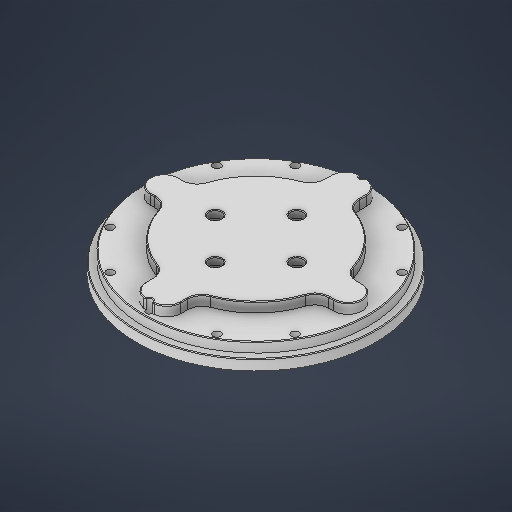
# Autodesk Inventor part: Build Plateform
Saved by Autodesk Inventor 2025 (Build 290162000, 162)
## iProperties
Created: 2024-08-23
Part Number: Build Plateform
Material: Generic
Document SubType Name: Modeling
Designer: mayhe
Density: 1 g/cm^3
Appearance: Default
Author: mayhe
Autodesk Inventor part; units mm, degrees
ref_plane "YZ Plane" through (0, 0, 0) normal (1, 0, 0) x (0, 1, 0)
ref_plane "XZ Plane" through (0, 0, 0) normal (0, 1, 0) x (-1, 0, 0)
ref_plane "XY Plane" through (0, 0, 0) normal (0, 0, 1) x (1, 0, 0)
sketch "Sketch1" plane through (0, 0, 0) normal (0, 1, 0) x (-1, 0, 0)
  circle A0 centre (0, 0) radius 85
  circle A1 centre (0, 0) radius 80
  circle A2 centre (0, 0) radius 76
  line L0 (65, 0) -> (65, 0)
  line L1 (-2.5, -76) -> (2.5, -76)
  line L2 (2.5, 76) -> (-2.5, 76)
  line L3 (-12.5, -76) -> (12.5, 76) construction
  line L4 (12.5, -76) -> (-12.5, 76) construction
  line L5 (-75.339233, 0) -> (-75.339233, 0)
  line L6 (75.339233, 0) -> (75.339233, 0)
  line L7 (75.339233, 10) -> (-75.339233, -10) construction
  line L8 (-75.339233, 10) -> (75.339233, -10) construction
  arc A3 (65.339233, -10) -> (75.339233, 0) centre (65.339233, 0) ccw
  arc A4 (75.339233, 0) -> (65.339233, 10) centre (65.339233, 0) ccw
  arc A5 (12.5, 66) -> (2.5, 76) centre (2.5, 66) ccw
  arc A6 (-2.5, 76) -> (-12.5, 66) centre (-2.5, 66) ccw
  arc A7 (2.5, -76) -> (12.5, -66) centre (2.5, -66) ccw
  arc A8 (-12.5, -66) -> (-2.5, -76) centre (-2.5, -66) ccw
  arc A9 (-75.339233, 0) -> (-65.339233, -10) centre (-65.339233, 0) ccw
  arc A10 (-65.339233, 10) -> (-75.339233, 0) centre (-65.339233, 0) ccw
  arc A11 (-52.331725, -16.923077) -> (-19.038462, -51.599777) centre (0, 0) ccw
  arc A12 (19.038462, -51.599777) -> (52.331725, -16.923077) centre (0, 0) ccw
  arc A13 (52.331725, 16.923077) -> (19.038462, 51.599777) centre (0, 0) ccw
  arc A14 (-19.038462, 51.599777) -> (-52.331725, 16.923077) centre (0, 0) ccw
  line L9 (12.5, -66) -> (12.5, -60.981555)
  line L10 (12.5, -1.659162) -> (12.5, 1.659162)
  line L11 (12.5, 60.981555) -> (12.5, 66)
  line L12 (-12.5, 66) -> (-12.5, 60.981555)
  line L13 (-12.5, -60.981555) -> (-12.5, -66)
  line L14 (-65.339233, -10) -> (-61.846584, -10)
  line L15 (61.846584, -10) -> (65.339233, -10)
  line L16 (65.339233, 10) -> (61.846584, 10)
  line L17 (-61.846584, 10) -> (-65.339233, 10)
  arc A15 (-12.5, -60.981555) -> (-19.038462, -51.599777) centre (-22.5, -60.981555) ccw
  arc A16 (-52.331725, -16.923077) -> (-61.846584, -10) centre (-61.846584, -20) ccw
  arc A17 (-61.846584, 10) -> (-52.331725, 16.923077) centre (-61.846584, 20) ccw
  arc A18 (-19.038462, 51.599777) -> (-12.5, 60.981555) centre (-22.5, 60.981555) ccw
  arc A19 (12.5, 60.981555) -> (19.038462, 51.599777) centre (22.5, 60.981555) ccw
  arc A20 (52.331725, 16.923077) -> (61.846584, 10) centre (61.846584, 20) ccw
  arc A21 (61.846584, -10) -> (52.331725, -16.923077) centre (61.846584, -20) ccw
  arc A22 (19.038462, -51.599777) -> (12.5, -60.981555) centre (22.5, -60.981555) ccw
  point P0 (-54.083269, 10)
  point P1 (-54.083269, -10)
  point P2 (-12.5, -53.560713)
  point P3 (12.5, -53.560713)
  point P4 (54.083269, -10)
  point P5 (54.083269, 10)
  point P6 (12.5, 53.560713)
  point P7 (-12.5, 53.560713)
  point P8 (3.918132, 75.898934)
  point P9 (-3.918132, 75.898934)
  point P10 (-3.918132, -75.898934)
  point P11 (3.918132, -75.898934)
  point P12 (75.339233, 0)
  point P13 (0, -76)
  point P14 (0, 76)
  dimension "d26" = 152
  dimension "d24" = 170
  dimension "d25" = 160
  dimension "d27" = 25
  dimension "d29" = 20
  dimension "d30" = 10
  dimension "d31" = 10
  dimension "d32" = 10
  constraints: 48 point on circle, 42 tangent, 36 end point, 22 centre point, 18 point on line, 13 equal radius, 12 parallel, 5 perpendicular, 4 midpoint, 3 coincident, 3 horizontal, 3 other
  measures "d24" diameter of A0
  measures "d25" diameter of A1
  measures "d27" distance of L4.end L3.end
  measures "d29" distance of L7.end L8.start
  measures "d30" radius of A3
  measures "d31" radius of A15
  measures "d32" radius of A18
extrude "Extrusion1" add sketch "Sketch1" along normal blind 21.5 contours A5 L11 A19 A13 A20 L16 A4 A3 L15 A21 A12 A22 L9 A7 A2 A8 L13 A15 A11 A16 L14 A9 A10 L17 A17 A14 A18 L12 A6
extrude "Extrusion2" add sketch "Sketch1" along normal blind 14.5 contours A1 | A2 A7 L9 A22 A12 A21 L15 A3 A4 L16 A20 A13 A19 L11 A5 | A2 L2 A5 | A7 L1 A2 | A2 A6 L2 | L1 A8 A2 | A6 L12 A18 A14 A17 L17 A10 A9 L14 A16 A11 A15 L13 A8 A2
extrude "Extrusion3" add sketch "Sketch1" along normal blind 7.5 contours A0
sketch "Sketch2" plane through (0, 21.5, 0) normal (0, 1, 0) x (1, 0, 0)
  circle A0 centre (0, 0) radius 29
  circle A1 centre (0, 29) radius 4.5
  circle A2 centre (0, 29) radius 2.5
  circle A3 centre (-29, 0) radius 4.5
  circle A4 centre (-29, 0) radius 2.5
  circle A5 centre (0, -29) radius 4.5
  circle A6 centre (0, -29) radius 2.5
  circle A7 centre (29, 0) radius 4.5
  circle A8 centre (29, 0) radius 2.5
  dimension "d40" = 58
  dimension "d41" = 9
  dimension "d42" = 5
  dimension "d45" = 360
  constraints: 8 centre point, 5 coincident, 1 vertical alignment, 19 other
  measures "d41" diameter of A1
  measures "d42" diameter of A2
extrude "Extrusion4" cut sketch "Sketch2" against normal blind 5 contours A0 A8 | A0 A8 | A8 A0 A7 | A0 A7 A8 | A1 A0 A2 | A0 A2 A1 | A5 A0 A6 | A0 A6 A5 | A2 A0 | A0 A2 | A6 A0 | A0 A6 | A3 A0 A4 | A0 A4 A3 | A4 A0 | A0 A4
hole "Hole1" at (29, 21.5, 0) at (0, 21.5, 29) at (-29, 21.5, 0) at (0, 21.5, -29) direction (0, -1, 0) diameter 5.5 end through all
sketch "Sketch3" plane through (0, 21.5, 0) normal (0, 1, 0) x (1, 0, 0)
  circle A0 centre (0, 0) radius 76
  circle A1 centre (0, 76) radius 1.75
  circle A2 centre (0, -76) radius 1.75
  dimension "d56" = 152
  dimension "d57" = 3.5
  dimension "d60" = 360
  constraints: 2 centre point, 1 coincident, 1 vertical alignment, 7 other
  measures "d57" diameter of A1
hole "Hole2" at (0, 21.5, -76) at (0, 21.5, 76) direction (0, -1, 0) diameter 4.5 end through all
sketch "Sketch4" plane through (0, 0, 0) normal (0, -1, 0) x (1, 0, 0)
  arc A0 (-19.364917, 35) -> (19.364917, 35) centre (0, 0) ccw
  line L0 (19.364917, 35) -> (-19.364917, 35)
  circle A1 centre (0, 0) radius 10
  dimension "d69" = 80
  dimension "d70" = 5
  dimension "d71" = 20
  constraints: 2 centre point, 2 coincident, 2 end point, 2 point on circle, 1 horizontal
  measures "d69" diameter of A0
  measures "d70" distance edge to line of A0 L0
  measures "d71" diameter of A1
extrude "Extrusion5" cut sketch "Sketch4" against normal blind 1.5
extrude "Extrusion6" cut sketch "Sketch4" against normal blind 12 contours A1
sketch "Sketch5" plane through (0, 14.5, 0) normal (0, 1, 0) x (1, 0, 0)
  circle A0 centre (0, 0) radius 10
  arc A1 (-2.249753, 75.966694) -> (2.249753, 75.966694) centre (0, 76) ccw
  circle A2 centre (0, 0) radius 76
  arc A3 (2.249753, -75.966694) -> (-2.249753, -75.966694) centre (0, -76) ccw
  circle A4 centre (0, -76) radius 2.5
  circle A5 centre (38, -65.817931) radius 2.5
  circle A6 centre (65.817931, -38) radius 2.5
  circle A7 centre (76, 0) radius 2.5
  circle A8 centre (65.817931, 38) radius 2.5
  circle A9 centre (38, 65.817931) radius 2.5
  circle A10 centre (0, 76) radius 2.5
  circle A11 centre (-38, 65.817931) radius 2.5
  circle A12 centre (-65.817931, 38) radius 2.5
  circle A13 centre (-76, 0) radius 2.5
  circle A14 centre (-65.817931, -38) radius 2.5
  circle A15 centre (-38, -65.817931) radius 2.5
  dimension "d76" = 5
  dimension "d79" = 360
  constraints: 13 centre point, 2 coincident, 1 point on circle, 25 other
  measures "d76" diameter of A4
hole "Hole3" at (-38, 14.5, 65.817931) at (-65.817931, 14.5, 38) at (-65.817931, 14.5, -38) at (-38, 14.5, -65.817931) at (38, 14.5, -65.817931) at (65.817931, 14.5, -38) at (65.817931, 14.5, 38) at (38, 14.5, 65.817931) direction (0, -1, 0) diameter 5.5 end through all
chamfer "Chamfer1" distance 0.5 angle 45 33 edges at (39.6742, 21.5, 38.0914) (55.9631, 21.5, 11.9139) (63.5929, 21.5, 10) (75.3392, 21.5, 0) (63.5929, 21.5, -10) (55.9631, 21.5, -11.9139) (39.6742, 21.5, -38.0914) (14.2959, 21.5, -55.2638) (12.5, 21.5, -63.4908) (10.0558, 21.5, -72.5505) (14.2959, 21.5, 55.2638) (12.5, 21.5, 63.4908) (10.0558, 21.5, 72.5505) (-14.2959, 21.5, 55.2638) (-12.5, 21.5, 63.4908) (-10.0558, 21.5, 72.5505) (-39.6742, 21.5, 38.0914) (-55.9631, 21.5, 11.9139) (-63.5929, 21.5, 10) (-75.3392, 21.5, 0) (-63.5929, 21.5, -10) (-55.9631, 21.5, -11.9139) (-39.6742, 21.5, -38.0914) (-14.2959, 21.5, -55.2638) (-12.5, 21.5, -63.4908) (-10.0558, 21.5, -72.5505) (-4.5, 21.5, 29) (-33.5, 21.5, 0) (-4.5, 21.5, -29) (24.5, 21.5, 0) (1.5792, 21.5, -74.3973) (-1.5792, 21.5, -74.3973) (0, 21.5, 73.75)
chamfer "Chamfer2" distance 0.5 angle 45 2 edges at (80, 14.5, 0) (85, 7.5, 0)
sketch "Sketch7" plane through (0, 21.5, 0) normal (0, 1, 0) x (1, 0, 0)
  circle A0 centre (0, 0) radius 47.5
  circle A1 centre (47.5, 0) radius 2.5
  circle A2 centre (43.884278, 18.177463) radius 2.5
  circle A3 centre (33.587572, 33.587572) radius 2.5
  circle A4 centre (18.177463, 43.884278) radius 2.5
  circle A5 centre (0, 47.5) radius 2.5
  circle A6 centre (-18.177463, 43.884278) radius 2.5
  circle A7 centre (-33.587572, 33.587572) radius 2.5
  circle A8 centre (-43.884278, 18.177463) radius 2.5
  circle A9 centre (-47.5, 0) radius 2.5
  circle A10 centre (-43.884278, -18.177463) radius 2.5
  circle A11 centre (-33.587572, -33.587572) radius 2.5
  circle A12 centre (-18.177463, -43.884278) radius 2.5
  circle A13 centre (0, -47.5) radius 2.5
  circle A14 centre (18.177463, -43.884278) radius 2.5
  circle A15 centre (33.587572, -33.587572) radius 2.5
  circle A16 centre (43.884278, -18.177463) radius 2.5
  dimension "d107" = 95
  dimension "d108" = 5
  dimension "d111" = 360
  constraints: 16 centre point, 1 coincident, 1 horizontal alignment, 35 other
  measures "d108" diameter of A1
hole "Hole5" [suppressed]
sketch "Sketch8" plane through (0, 0, 0) normal (0, -1, 0) x (1, 0, 0)
  circle A0 centre (38, -65.817931) radius 2.75
  circle A1 centre (0, -29) radius 2.75
  circle A2 centre (38, 65.817931) radius 2.75
  circle A3 centre (38, 65.817931) radius 3.875
  circle A4 centre (65.817931, 38) radius 2.75
  circle A5 centre (65.817931, 38) radius 3.875
  circle A6 centre (65.817931, -38) radius 2.75
  circle A7 centre (65.817931, -38) radius 3.875
  circle A8 centre (38, -65.817931) radius 3.875
  circle A9 centre (0, -76) radius 2.25
  circle A10 centre (-38, -65.817931) radius 2.75
  circle A11 centre (-38, -65.817931) radius 3.875
  circle A12 centre (-65.817931, -38) radius 2.75
  circle A13 centre (-65.817931, -38) radius 3.875
  circle A14 centre (-65.817931, 38) radius 2.75
  circle A15 centre (-65.817931, 38) radius 3.875
  circle A16 centre (-38, 65.817931) radius 2.75
  circle A17 centre (-38, 65.817931) radius 3.875
  circle A18 centre (29, 0) radius 2.75
  circle A19 centre (29, 0) radius 3.875
  circle A20 centre (0, -29) radius 3.875
  circle A21 centre (-29, 0) radius 2.75
  circle A22 centre (-29, 0) radius 3.875
  circle A23 centre (0, 29) radius 2.75
  circle A24 centre (0, 29) radius 3.875
  circle A25 centre (0, 76) radius 2.25
  circle A26 centre (0, 76) radius 3.625
  circle A27 centre (0, -76) radius 3.625
  line L0 (69.705483, 35.784651) -> (65.843159, 33.525607)
  line L1 (65.843159, 33.525607) -> (61.955606, 35.740955)
  line L2 (61.955606, 35.740955) -> (61.930378, 40.215349)
  line L3 (61.930378, 40.215349) -> (65.792703, 42.474393)
  line L4 (65.792703, 42.474393) -> (69.680255, 40.259045)
  line L5 (69.680255, 40.259045) -> (69.705483, 35.784651)
  line L6 (61.943019, -35.762615) -> (65.818107, -33.525535)
  line L7 (65.818107, -33.525535) -> (69.693019, -35.76292)
  line L8 (69.693019, -35.76292) -> (69.692843, -40.237385)
  line L9 (69.692843, -40.237385) -> (65.817755, -42.474465)
  line L10 (65.817755, -42.474465) -> (61.942843, -40.23708)
  line L11 (61.942843, -40.23708) -> (61.943019, -35.762615)
  line L12 (34.125, -63.580698) -> (38, -61.343466)
  line L13 (38, -61.343466) -> (41.875, -63.580698)
  line L14 (41.875, -63.580698) -> (41.875, -68.055163)
  line L15 (41.875, -68.055163) -> (38, -70.292395)
  line L16 (38, -70.292395) -> (34.125, -68.055163)
  line L17 (34.125, -68.055163) -> (34.125, -63.580698)
  line L18 (-3.606269, -73.874992) -> (0.037176, -71.814376)
  line L19 (0.037176, -71.814376) -> (3.643445, -73.939384)
  line L20 (3.643445, -73.939384) -> (3.606269, -78.125008)
  line L21 (3.606269, -78.125008) -> (-0.037176, -80.185624)
  line L22 (-0.037176, -80.185624) -> (-3.643445, -78.060616)
  line L23 (-3.643445, -78.060616) -> (-3.606269, -73.874992)
  line L24 (-41.875, -63.580698) -> (-38, -61.343466)
  line L25 (-38, -61.343466) -> (-34.125, -63.580698)
  line L26 (-34.125, -63.580698) -> (-34.125, -68.055163)
  line L27 (-34.125, -68.055163) -> (-38, -70.292395)
  line L28 (-38, -70.292395) -> (-41.875, -68.055163)
  line L29 (-41.875, -68.055163) -> (-41.875, -63.580698)
  line L30 (-69.692845, -35.76262) -> (-65.81776, -33.525535)
  line L31 (-65.81776, -33.525535) -> (-61.942845, -35.762916)
  line L32 (-61.942845, -35.762916) -> (-61.943016, -40.23738)
  line L33 (-61.943016, -40.23738) -> (-65.818101, -42.474465)
  line L34 (-65.818101, -42.474465) -> (-69.693016, -40.237084)
  line L35 (-69.693016, -40.237084) -> (-69.692845, -35.76262)
  line L36 (-69.776476, 40.085846) -> (-65.990807, 42.471124)
  line L37 (-65.990807, 42.471124) -> (-62.032262, 40.385278)
  line L38 (-62.032262, 40.385278) -> (-61.859386, 35.914154)
  line L39 (-61.859386, 35.914154) -> (-65.645054, 33.528876)
  line L40 (-65.645054, 33.528876) -> (-69.603599, 35.614722)
  line L41 (-69.603599, 35.614722) -> (-69.776476, 40.085846)
  line L42 (-41.875, 68.055163) -> (-38, 70.292395)
  line L43 (-38, 70.292395) -> (-34.125, 68.055163)
  line L44 (-34.125, 68.055163) -> (-34.125, 63.580698)
  line L45 (-34.125, 63.580698) -> (-38, 61.343466)
  line L46 (-38, 61.343466) -> (-41.875, 63.580698)
  line L47 (-41.875, 63.580698) -> (-41.875, 68.055163)
  line L48 (-3.675534, 78.002819) -> (-0.103274, 80.184515)
  line L49 (-0.103274, 80.184515) -> (3.572259, 78.181696)
  line L50 (3.572259, 78.181696) -> (3.675534, 73.997181)
  line L51 (3.675534, 73.997181) -> (0.103274, 71.815485)
  line L52 (0.103274, 71.815485) -> (-3.572259, 73.818304)
  line L53 (-3.572259, 73.818304) -> (-3.675534, 78.002819)
  line L54 (34.125, 68.055163) -> (38, 70.292395)
  line L55 (38, 70.292395) -> (41.875, 68.055163)
  line L56 (41.875, 68.055163) -> (41.875, 63.580698)
  line L57 (41.875, 63.580698) -> (38, 61.343466)
  line L58 (38, 61.343466) -> (34.125, 63.580698)
  line L59 (34.125, 63.580698) -> (34.125, 68.055163)
  line L60 (25.125, 2.237232) -> (29, 4.474465)
  line L61 (29, 4.474465) -> (32.875, 2.237232)
  line L62 (32.875, 2.237232) -> (32.875, -2.237232)
  line L63 (32.875, -2.237232) -> (29, -4.474465)
  line L64 (29, -4.474465) -> (25.125, -2.237232)
  line L65 (25.125, -2.237232) -> (25.125, 2.237232)
  line L66 (2.341169, 32.813104) -> (4.472829, 28.87904)
  line L67 (4.472829, 28.87904) -> (2.13166, 25.065936)
  line L68 (2.13166, 25.065936) -> (-2.341169, 25.186896)
  line L69 (-2.341169, 25.186896) -> (-4.472829, 29.12096)
  line L70 (-4.472829, 29.12096) -> (-2.13166, 32.934064)
  line L71 (-2.13166, 32.934064) -> (2.341169, 32.813104)
  line L72 (-32.875, 2.237232) -> (-29, 4.474465)
  line L73 (-29, 4.474465) -> (-25.125, 2.237232)
  line L74 (-25.125, 2.237232) -> (-25.125, -2.237232)
  line L75 (-25.125, -2.237232) -> (-29, -4.474465)
  line L76 (-29, -4.474465) -> (-32.875, -2.237232)
  line L77 (-32.875, -2.237232) -> (-32.875, 2.237232)
  line L78 (-2.237232, -32.875) -> (-4.474465, -29)
  line L79 (-4.474465, -29) -> (-2.237232, -25.125)
  line L80 (-2.237232, -25.125) -> (2.237232, -25.125)
  line L81 (2.237232, -25.125) -> (4.474465, -29)
  line L82 (4.474465, -29) -> (2.237232, -32.875)
  line L83 (2.237232, -32.875) -> (-2.237232, -32.875)
  circle A28 centre (0, 29) radius 2.75
  point P0 (0, 0)
  point P1 (0, 0)
  point P2 (69.692869, 38.021848)
  point P3 (61.942931, -37.999847)
  point P4 (34.125, -65.817931)
  point P5 (-3.624857, -75.967804)
  point P6 (-41.875, -65.817931)
  point P7 (-69.692931, -37.999852)
  point P8 (-69.690037, 37.850284)
  point P9 (-41.875, 65.817931)
  point P10 (-3.623896, 75.910562)
  point P11 (34.125, 65.817931)
  point P12 (25.125, 0)
  point P13 (0.104754, 32.873584)
  point P14 (-32.875, 0)
  point P15 (0, -32.875)
  point P16 (39.905469, 2.748375)
  point P17 (39.905469, -2.748375)
  dimension "d120" = 7.75
  dimension "d121" = 7.75
  dimension "d122" = 7.75
  dimension "d123" = 7.75
  dimension "d125" = 7.75
  dimension "d126" = 7.75
  dimension "d127" = 7.75
  dimension "d128" = 7.75
  dimension "d129" = 7.75
  dimension "d130" = 7.75
  dimension "d131" = 7.75
  dimension "d132" = 7.75
  dimension "d133" = 7.25
  dimension "d134" = 7.25
  constraints: 168 end point, 28 coincident, 14 midpoint, 6 horizontal alignment, 3 point on line, 1 centre point, 1 concentric, 1 vertical alignment, 218 other
extrude "Extrusion7" cut sketch "Sketch8" against normal blind 4 contours A3 | L56 L57 A3 | A3 L55 L56 | A3 L54 L55 | L57 L58 A3 | A3 L59 L54 | L58 L59 A3 | A5 | L5 L0 A5 | A5 L4 L5 | A5 L3 L4 | L0 L1 A5 | A5 L2 L3 | L1 L2 A5 | A7 | L8 L9 A7 | A7 L7 L8 | A7 L6 L7 | L9 L10 A7 | A7 L11 L6 | L10 L11 A7 | A8 | L14 L15 A8 | A8 L13 L14 | A8 L12 L13 | L15 L16 A8 | A8 L17 L12 | L16 L17 A8 | A11 | L26 L27 A11 | A11 L25 L26 | A11 L24 L25 | L27 L28 A11 | A11 L29 L24 | L28 L29 A11 | A13 | L32 L33 A13 | A13 L31 L32 | A13 L30 L31 | L33 L34 A13 | A13 L35 L30 | L34 L35 A13 | A15 | A15 L38 L39 | A15 L37 L38 | L39 L40 A15 | A15 L36 L37 | L40 L41 A15 | A15 L41 L36 | A17 | L44 L45 A17 | A17 L43 L44 | A17 L42 L43 | L45 L46 A17 | A17 L47 L42 | L46 L47 A17 | A18 | A19 | L62 L63 A19 | A19 L61 L62 | A19 L60 L61 | L63 L64 A19 | A19 L65 L60 | L64 L65 A19 | A20 | A20 L81 L82 | A20 L80 L81 | L82 L83 A20 | A20 L79 L80 | L83 L78 A20 | A20 L78 L79 | A22 | L74 L75 A22 | A22 L73 L74 | A22 L72 L73 | L75 L76 A22 | A22 L77 L72 | L76 L77 A22 | A24 | A24 L66 L67 | A24 L71 L66 | L67 L68 A24 | A24 L70 L71 | L68 L69 A24 | A24 L69 L70
extrude "Extrusion8" cut sketch "Sketch8" against normal blind 3.5 contours A26 | L50 L51 A26 | A26 L49 L50 | A26 L48 L49 | L51 L52 A26 | A26 L53 L48 | L52 L53 A26 | A27 | L20 L21 A27 | A27 L19 L20 | A27 L18 L19 | L21 L22 A27 | A27 L23 L18 | L22 L23 A27
body "Solid1"
